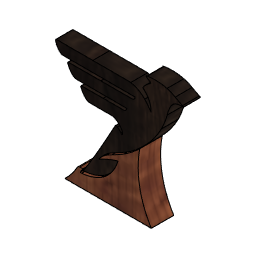
BlackSwiftDeskLogo v10 (Autodesk Fusion 360 design; units mm, degrees)
Autodesk Fusion 360 part; units mm, degrees
sketch "Sketch1" plane through (0, 0, 0) normal (0, 1, 0) x (1, 0, 0)
  spline S0 degree 3 poles (28.812599, -0.914385) (28.812599, -1.007661) (29.30972, -1.834065) (29.917311, -2.750838) knots 0 0 0 0 1 1 1 1
  spline S1 degree 3 poles (29.917311, -2.750838) (36.944588, -13.354057) (46.936102, -30.456433) (58.618766, -51.878822) knots 0 0 0 0 1 1 1 1
  spline S2 degree 3 poles (58.618766, -51.878822) (60.219164, -54.813461) (61.65408, -57.379058) (61.807463, -57.580155) knots 0 0 0 0 1 1 1 1
  spline S3 degree 3 poles (61.807463, -57.580155) (62.243331, -58.151604) (62.6887, -58.094845) (63.845395, -57.320437) knots 0 0 0 0 1 1 1 1
  spline S4 degree 3 poles (63.845395, -57.320437) (64.951702, -56.579755) (66.160509, -55.405523) (67.347976, -53.918028) knots 0 0 0 0 1 1 1 1
  spline S5 degree 3 poles (67.347976, -53.918028) (68.302152, -52.722769) (68.569408, -52.552013) (68.881908, -52.937928) knots 0 0 0 0 1 1 1 1
  spline S6 degree 3 poles (68.881908, -52.937928) (69.341546, -53.505563) (69.008645, -55.565192) (68.194272, -57.192261) knots 0 0 0 0 1 1 1 1
  spline S7 degree 3 poles (68.194272, -57.192261) (67.571278, -58.436976) (66.865745, -59.388616) (65.693126, -60.565893) knots 0 0 0 0 1 1 1 1
  spline S8 degree 3 poles (65.693126, -60.565893) (63.643539, -62.623611) (61.536026, -63.942213) (59.43194, -64.483299) knots 0 0 0 0 1 1 1 1
  spline S9 degree 3 poles (59.43194, -64.483299) (58.739509, -64.661363) (57.820927, -64.673156) (47.446235, -64.637132) knots 0 0 0 0 1 1 1 1
  spline S10 degree 3 poles (47.446235, -64.637132) (36.109744, -64.597772) (34.64539, -64.636087) (33.594249, -64.998073) knots 0 0 0 0 1 1 1 1
  spline S11 degree 3 poles (33.594249, -64.998073) (32.71821, -65.299894) (31.855594, -65.916002) (30.696252, -67.067923) knots 0 0 0 0 1 1 1 1
  spline S12 degree 3 poles (30.696252, -67.067923) (29.044949, -68.708652) (27.40767, -71.223347) (26.483234, -73.538694) knots 0 0 0 0 1 1 1 1
  spline S13 degree 3 poles (26.483234, -73.538694) (26.080684, -74.546929) (26.054861, -74.963611) (26.376872, -75.25504) knots 0 0 0 0 1 1 1 1
  spline S14 degree 3 poles (26.376872, -75.25504) (26.605076, -75.461575) (27.181933, -75.468375) (49.063672, -75.522586) knots 0 0 0 0 1 1 1 1
  line L0 (49.063672, -75.522586) -> (71.516311, -75.57821)
  line L1 (71.516311, -75.57821) -> (71.87243, -75.911946)
  spline S15 degree 3 poles (71.87243, -75.911946) (72.373465, -76.381488) (73.310826, -77.836591) (73.310826, -78.144823) knots 0 0 0 0 1 1 1 1
  spline S16 degree 3 poles (73.310826, -78.144823) (73.310826, -78.286466) (73.199567, -78.480283) (73.063583, -78.57553) knots 0 0 0 0 1 1 1 1
  spline S17 degree 3 poles (73.063583, -78.57553) (72.841591, -78.731021) (70.208488, -78.749104) (47.282424, -78.752587) knots 0 0 0 0 1 1 1 1
  spline S18 degree 3 poles (47.282424, -78.752587) (25.94621, -78.755716) (21.60542, -78.781964) (20.878127, -78.911613) knots 0 0 0 0 1 1 1 1
  spline S19 degree 3 poles (20.878127, -78.911613) (18.537316, -79.328857) (16.127566, -81.699245) (14.031978, -85.645935) knots 0 0 0 0 1 1 1 1
  spline S20 degree 3 poles (14.031978, -85.645935) (12.729457, -88.099011) (12.388433, -89.429148) (12.986959, -89.721938) knots 0 0 0 0 1 1 1 1
  spline S21 degree 3 poles (12.986959, -89.721938) (13.094562, -89.774576) (28.25081, -89.842673) (46.667514, -89.873265) knots 0 0 0 0 1 1 1 1
  spline S22 degree 3 poles (46.667514, -89.873265) (73.988945, -89.918649) (80.199445, -89.955709) (80.407863, -90.074607) knots 0 0 0 0 1 1 1 1
  spline S23 degree 3 poles (80.407863, -90.074607) (80.695616, -90.238763) (81.565868, -91.378616) (81.893942, -92.021069) knots 0 0 0 0 1 1 1 1
  spline S24 degree 3 poles (81.893942, -92.021069) (82.160264, -92.542607) (82.084297, -92.821555) (81.633093, -92.978844) knots 0 0 0 0 1 1 1 1
  spline S25 degree 3 poles (81.633093, -92.978844) (81.387485, -93.064463) (70.631073, -93.099389) (44.504993, -93.099389) knots 0 0 0 0 1 1 1 1
  spline S26 degree 3 poles (44.504993, -93.099389) (3.876362, -93.099389) (7.079301, -93.041478) (5.789219, -93.799384) knots 0 0 0 0 1 1 1 1
  spline S27 degree 3 poles (5.789219, -93.799384) (4.940553, -94.297963) (3.299284, -95.96935) (2.48931, -97.15985) knots 0 0 0 0 1 1 1 1
  spline S28 degree 3 poles (2.48931, -97.15985) (1.193036, -99.065112) (0.103075, -101.631647) (0.094025, -102.800034) knots 0 0 0 0 1 1 1 1
  spline S29 degree 3 poles (0.094025, -102.800034) (0.090443, -103.262371) (0.141743, -103.415042) (0.381101, -103.654396) knots 0 0 0 0 1 1 1 1
  line L2 (0.381101, -103.654396) -> (0.672538, -103.94583)
  line L3 (0.672538, -103.94583) -> (38.465688, -103.94583)
  spline S30 degree 3 poles (38.465688, -103.94583) (74.521314, -103.94583) (76.315092, -103.936495) (77.482534, -103.742926) knots 0 0 0 0 1 1 1 1
  spline S31 degree 3 poles (77.482534, -103.742926) (83.17461, -102.799111) (87.481522, -100.516999) (91.89345, -96.106981) knots 0 0 0 0 1 1 1 1
  spline S32 degree 3 poles (91.89345, -96.106981) (94.083858, -93.917523) (95.823661, -91.737445) (97.489688, -89.094547) knots 0 0 0 0 1 1 1 1
  line L4 (97.489688, -89.094547) -> (98.366273, -87.703977)
  line L5 (98.366273, -87.703977) -> (98.305674, -89.650774)
  spline S33 degree 3 poles (98.305674, -89.650774) (98.239918, -91.763348) (98.039913, -92.960782) (97.43434, -94.867524) knots 0 0 0 0 1 1 1 1
  spline S34 degree 3 poles (97.43434, -94.867524) (97.05087, -96.074941) (96.056162, -98.221095) (95.340677, -99.384761) knots 0 0 0 0 1 1 1 1
  spline S35 degree 3 poles (95.340677, -99.384761) (94.230244, -101.190765) (92.524316, -103.150251) (90.91543, -104.467741) knots 0 0 0 0 1 1 1 1
  spline S36 degree 3 poles (90.91543, -104.467741) (90.275302, -104.991935) (90.108897, -105.190363) (90.108897, -105.429509) knots 0 0 0 0 1 1 1 1
  spline S37 degree 3 poles (90.108897, -105.429509) (90.108897, -106.16981) (91.997399, -108.567541) (93.735112, -110.033524) knots 0 0 0 0 1 1 1 1
  spline S38 degree 3 poles (93.735112, -110.033524) (94.222711, -110.444874) (95.270794, -111.221163) (96.064182, -111.758612) knots 0 0 0 0 1 1 1 1
  spline S39 degree 3 poles (96.064182, -111.758612) (97.206454, -112.532395) (97.551062, -112.826473) (97.71977, -113.171449) knots 0 0 0 0 1 1 1 1
  spline S40 degree 3 poles (97.71977, -113.171449) (97.929662, -113.600668) (97.929662, -113.612985) (97.71977, -114.005009) knots 0 0 0 0 1 1 1 1
  spline S41 degree 3 poles (97.71977, -114.005009) (97.54598, -114.329584) (97.285577, -114.515665) (96.306698, -115.014762) knots 0 0 0 0 1 1 1 1
  spline S42 degree 3 poles (96.306698, -115.014762) (95.039089, -115.661068) (94.193281, -116.31074) (93.658715, -117.048689) knots 0 0 0 0 1 1 1 1
  spline S43 degree 3 poles (93.658715, -117.048689) (93.117943, -117.795204) (93.162979, -117.844139) (94.586522, -118.05692) knots 0 0 0 0 1 1 1 1
  spline S44 degree 3 poles (94.586522, -118.05692) (101.519329, -119.09318) (108.735231, -118.782906) (114.86716, -117.184877) knots 0 0 0 0 1 1 1 1
  spline S45 degree 3 poles (114.86716, -117.184877) (117.554906, -116.484431) (119.695907, -115.590846) (123.298495, -113.665903) knots 0 0 0 0 1 1 1 1
  spline S46 degree 3 poles (123.298495, -113.665903) (127.961824, -111.174193) (129.500391, -110.372518) (130.744363, -109.78622) knots 0 0 0 0 1 1 1 1
  spline S47 degree 3 poles (130.744363, -109.78622) (131.458373, -109.449702) (132.043895, -109.144521) (132.045518, -109.10804) knots 0 0 0 0 1 1 1 1
  spline S48 degree 3 poles (132.045518, -109.10804) (132.047258, -109.071559) (131.287841, -109.007388) (130.358188, -108.965437) knots 0 0 0 0 1 1 1 1
  spline S49 degree 3 poles (130.358188, -108.965437) (124.388559, -108.696058) (121.480194, -107.39743) (119.240974, -104.001451) knots 0 0 0 0 1 1 1 1
  spline S50 degree 3 poles (119.240974, -104.001451) (117.657667, -101.600224) (116.596502, -98.956061) (115.040811, -93.535774) knots 0 0 0 0 1 1 1 1
  spline S51 degree 3 poles (115.040811, -93.535774) (113.32995, -87.574855) (111.543148, -83.000167) (109.026252, -78.136858) knots 0 0 0 0 1 1 1 1
  spline S52 degree 3 poles (109.026252, -78.136858) (104.535546, -69.459641) (98.796243, -61.728751) (91.22576, -54.159483) knots 0 0 0 0 1 1 1 1
  spline S53 degree 3 poles (91.22576, -54.159483) (85.617623, -48.552238) (79.732979, -43.799887) (73.340409, -39.715556) knots 0 0 0 0 1 1 1 1
  spline S54 degree 3 poles (73.340409, -39.715556) (70.30336, -37.775133) (67.906625, -36.437854) (60.851314, -32.747182) knots 0 0 0 0 1 1 1 1
  spline S55 degree 3 poles (60.851314, -32.747182) (57.635155, -31.064785) (56.324494, -30.311792) (54.677187, -29.200059) knots 0 0 0 0 1 1 1 1
  spline S56 degree 3 poles (54.677187, -29.200059) (51.971909, -27.37431) (49.870008, -25.48514) (48.476813, -23.627214) knots 0 0 0 0 1 1 1 1
  spline S57 degree 3 poles (48.476813, -23.627214) (47.732466, -22.634575) (47.07678, -21.511506) (47.180841, -21.40744) knots 0 0 0 0 1 1 1 1
  spline S58 degree 3 poles (47.180841, -21.40744) (47.215665, -21.37261) (47.690109, -21.60197) (48.235162, -21.917117) knots 0 0 0 0 1 1 1 1
  spline S59 degree 3 poles (48.235162, -21.917117) (52.504268, -24.385507) (58.551397, -27.044152) (64.046471, -28.868649) knots 0 0 0 0 1 1 1 1
  spline S60 degree 3 poles (64.046471, -28.868649) (66.31813, -29.622889) (66.858579, -29.77155) (66.858579, -29.642166) knots 0 0 0 0 1 1 1 1
  spline S61 degree 3 poles (66.858579, -29.642166) (66.858579, -29.459655) (65.725346, -26.393405) (65.272588, -25.350849) knots 0 0 0 0 1 1 1 1
  spline S62 degree 3 poles (65.272588, -25.350849) (63.047403, -20.227007) (60.46569, -16.387494) (56.741138, -12.662942) knots 0 0 0 0 1 1 1 1
  spline S63 degree 3 poles (56.741138, -12.662942) (54.272096, -10.193894) (52.293622, -8.639115) (49.369116, -6.869617) knots 0 0 0 0 1 1 1 1
  spline S64 degree 3 poles (49.369116, -6.869617) (43.741178, -3.464391) (36.717991, -1.281855) (29.897239, -0.818488) knots 0 0 0 0 1 1 1 1
  spline S65 degree 3 poles (29.897239, -0.818488) (28.967337, -0.75531) (28.812594, -0.768996) (28.812599, -0.914385) knots 0 0 0 0 1 1 1 1
extrude "Extrude1" add sketch "Sketch1" along normal blind 17.31645 makes body 1
sketch "Sketch2" plane through (0, 17.31645, 0) normal (0, 1, 0) x (-1, 0, 0)
  spline S0 degree 3 poles (-29.897239, 0.818488) (-28.967337, 0.75531) (-28.812594, 0.768996) (-28.812599, 0.914385) knots 0 0 0 0 1 1 1 1
  spline S1 degree 3 poles (-28.812599, 0.914385) (-28.812599, 1.007661) (-29.30972, 1.834065) (-29.917311, 2.750838) knots 0 0 0 0 1 1 1 1
  spline S2 degree 3 poles (-29.917311, 2.750838) (-36.944588, 13.354057) (-46.936102, 30.456433) (-58.618766, 51.878822) knots 0 0 0 0 1 1 1 1
  spline S3 degree 3 poles (-58.618766, 51.878822) (-60.219164, 54.813461) (-61.65408, 57.379058) (-61.807463, 57.580155) knots 0 0 0 0 1 1 1 1
  spline S4 degree 3 poles (-61.807463, 57.580155) (-62.243331, 58.151604) (-62.6887, 58.094845) (-63.845395, 57.320437) knots 0 0 0 0 1 1 1 1
  spline S5 degree 3 poles (-63.845395, 57.320437) (-64.951702, 56.579755) (-66.160509, 55.405523) (-67.347976, 53.918028) knots 0 0 0 0 1 1 1 1
  spline S6 degree 3 poles (-67.347976, 53.918028) (-68.302152, 52.722769) (-68.569408, 52.552013) (-68.881908, 52.937928) knots 0 0 0 0 1 1 1 1
  spline S7 degree 3 poles (-68.881908, 52.937928) (-69.341546, 53.505563) (-69.008645, 55.565192) (-68.194272, 57.192261) knots 0 0 0 0 1 1 1 1
  spline S8 degree 3 poles (-68.194272, 57.192261) (-67.571278, 58.436976) (-66.865745, 59.388616) (-65.693126, 60.565893) knots 0 0 0 0 1 1 1 1
  spline S9 degree 3 poles (-65.693126, 60.565893) (-63.643539, 62.623611) (-61.536026, 63.942213) (-59.43194, 64.483299) knots 0 0 0 0 1 1 1 1
  spline S10 degree 3 poles (-59.43194, 64.483299) (-58.739509, 64.661363) (-57.820927, 64.673156) (-47.446235, 64.637132) knots 0 0 0 0 1 1 1 1
  spline S11 degree 3 poles (-47.446235, 64.637132) (-36.109744, 64.597772) (-34.64539, 64.636087) (-33.594249, 64.998073) knots 0 0 0 0 1 1 1 1
  spline S12 degree 3 poles (-33.594249, 64.998073) (-32.71821, 65.299894) (-31.855594, 65.916002) (-30.696252, 67.067923) knots 0 0 0 0 1 1 1 1
  spline S13 degree 3 poles (-30.696252, 67.067923) (-29.044949, 68.708652) (-27.40767, 71.223347) (-26.483234, 73.538694) knots 0 0 0 0 1 1 1 1
  spline S14 degree 3 poles (-26.483234, 73.538694) (-26.080684, 74.546929) (-26.054861, 74.963611) (-26.376872, 75.25504) knots 0 0 0 0 1 1 1 1
  spline S15 degree 3 poles (-26.376872, 75.25504) (-26.605076, 75.461575) (-27.181933, 75.468375) (-49.063672, 75.522586) knots 0 0 0 0 1 1 1 1
  line L0 (-49.063672, 75.522586) -> (-71.516311, 75.57821)
  line L1 (-71.516311, 75.57821) -> (-71.87243, 75.911946)
  spline S16 degree 3 poles (-71.87243, 75.911946) (-72.373465, 76.381488) (-73.310826, 77.836591) (-73.310826, 78.144823) knots 0 0 0 0 1 1 1 1
  spline S17 degree 3 poles (-73.310826, 78.144823) (-73.310826, 78.286466) (-73.199567, 78.480283) (-73.063583, 78.57553) knots 0 0 0 0 1 1 1 1
  spline S18 degree 3 poles (-73.063583, 78.57553) (-72.841591, 78.731021) (-70.208488, 78.749104) (-47.282424, 78.752587) knots 0 0 0 0 1 1 1 1
  spline S19 degree 3 poles (-47.282424, 78.752587) (-25.94621, 78.755716) (-21.60542, 78.781964) (-20.878127, 78.911613) knots 0 0 0 0 1 1 1 1
  spline S20 degree 3 poles (-20.878127, 78.911613) (-18.537316, 79.328857) (-16.127566, 81.699245) (-14.031978, 85.645935) knots 0 0 0 0 1 1 1 1
  spline S21 degree 3 poles (-14.031978, 85.645935) (-12.729457, 88.099011) (-12.388433, 89.429148) (-12.986959, 89.721938) knots 0 0 0 0 1 1 1 1
  spline S22 degree 3 poles (-12.986959, 89.721938) (-13.094562, 89.774576) (-28.25081, 89.842673) (-46.667514, 89.873265) knots 0 0 0 0 1 1 1 1
  spline S23 degree 3 poles (-46.667514, 89.873265) (-73.988945, 89.918649) (-80.199445, 89.955709) (-80.407863, 90.074607) knots 0 0 0 0 1 1 1 1
  spline S24 degree 3 poles (-80.407863, 90.074607) (-80.695616, 90.238763) (-81.565868, 91.378616) (-81.893942, 92.021069) knots 0 0 0 0 1 1 1 1
  spline S25 degree 3 poles (-81.893942, 92.021069) (-82.160264, 92.542607) (-82.084297, 92.821555) (-81.633093, 92.978844) knots 0 0 0 0 1 1 1 1
  spline S26 degree 3 poles (-81.633093, 92.978844) (-81.387485, 93.064463) (-70.631073, 93.099389) (-44.504993, 93.099389) knots 0 0 0 0 1 1 1 1
  spline S27 degree 3 poles (-44.504993, 93.099389) (-3.876362, 93.099389) (-7.079301, 93.041478) (-5.789219, 93.799384) knots 0 0 0 0 1 1 1 1
  spline S28 degree 3 poles (-5.789219, 93.799384) (-4.940553, 94.297963) (-3.299284, 95.96935) (-2.48931, 97.15985) knots 0 0 0 0 1 1 1 1
  spline S29 degree 3 poles (-2.48931, 97.15985) (-1.193036, 99.065112) (-0.103075, 101.631647) (-0.094025, 102.800034) knots 0 0 0 0 1 1 1 1
  spline S30 degree 3 poles (-0.094025, 102.800034) (-0.090443, 103.262371) (-0.141743, 103.415042) (-0.381101, 103.654396) knots 0 0 0 0 1 1 1 1
  line L2 (-0.381101, 103.654396) -> (-0.672538, 103.94583)
  line L3 (-0.672538, 103.94583) -> (-38.465688, 103.94583)
  spline S31 degree 3 poles (-38.465688, 103.94583) (-74.521314, 103.94583) (-76.315092, 103.936495) (-77.482534, 103.742926) knots 0 0 0 0 1 1 1 1
  spline S32 degree 3 poles (-77.482534, 103.742926) (-83.17461, 102.799111) (-87.481522, 100.516999) (-91.89345, 96.106981) knots 0 0 0 0 1 1 1 1
  spline S33 degree 3 poles (-91.89345, 96.106981) (-94.083858, 93.917523) (-95.823661, 91.737445) (-97.489688, 89.094547) knots 0 0 0 0 1 1 1 1
  line L4 (-97.489688, 89.094547) -> (-98.366273, 87.703977)
  line L5 (-98.366273, 87.703977) -> (-98.305674, 89.650774)
  spline S34 degree 3 poles (-98.305674, 89.650774) (-98.239918, 91.763348) (-98.039913, 92.960782) (-97.43434, 94.867524) knots 0 0 0 0 1 1 1 1
  spline S35 degree 3 poles (-97.43434, 94.867524) (-97.05087, 96.074941) (-96.056162, 98.221095) (-95.340677, 99.384761) knots 0 0 0 0 1 1 1 1
  spline S36 degree 3 poles (-95.340677, 99.384761) (-94.230244, 101.190765) (-92.524316, 103.150251) (-90.91543, 104.467741) knots 0 0 0 0 1 1 1 1
  spline S37 degree 3 poles (-90.91543, 104.467741) (-90.275302, 104.991935) (-90.108897, 105.190363) (-90.108897, 105.429509) knots 0 0 0 0 1 1 1 1
  spline S38 degree 3 poles (-90.108897, 105.429509) (-90.108897, 106.16981) (-91.997399, 108.567541) (-93.735112, 110.033524) knots 0 0 0 0 1 1 1 1
  spline S39 degree 3 poles (-93.735112, 110.033524) (-94.222711, 110.444874) (-95.270794, 111.221163) (-96.064182, 111.758612) knots 0 0 0 0 1 1 1 1
  spline S40 degree 3 poles (-96.064182, 111.758612) (-97.206454, 112.532395) (-97.551062, 112.826473) (-97.71977, 113.171449) knots 0 0 0 0 1 1 1 1
  spline S41 degree 3 poles (-97.71977, 113.171449) (-97.929662, 113.600668) (-97.929662, 113.612985) (-97.71977, 114.005009) knots 0 0 0 0 1 1 1 1
  spline S42 degree 3 poles (-97.71977, 114.005009) (-97.54598, 114.329584) (-97.285577, 114.515665) (-96.306698, 115.014762) knots 0 0 0 0 1 1 1 1
  spline S43 degree 3 poles (-96.306698, 115.014762) (-95.039089, 115.661068) (-94.193281, 116.31074) (-93.658715, 117.048689) knots 0 0 0 0 1 1 1 1
  spline S44 degree 3 poles (-93.658715, 117.048689) (-93.117943, 117.795204) (-93.162979, 117.844139) (-94.586522, 118.05692) knots 0 0 0 0 1 1 1 1
  spline S45 degree 3 poles (-94.586522, 118.05692) (-101.519329, 119.09318) (-108.735231, 118.782906) (-114.86716, 117.184877) knots 0 0 0 0 1 1 1 1
  spline S46 degree 3 poles (-114.86716, 117.184877) (-117.554906, 116.484431) (-119.695907, 115.590846) (-123.298495, 113.665903) knots 0 0 0 0 1 1 1 1
  spline S47 degree 3 poles (-123.298495, 113.665903) (-127.961824, 111.174193) (-129.500391, 110.372518) (-130.744363, 109.78622) knots 0 0 0 0 1 1 1 1
  spline S48 degree 3 poles (-130.744363, 109.78622) (-131.458373, 109.449702) (-132.043895, 109.144521) (-132.045518, 109.10804) knots 0 0 0 0 1 1 1 1
  spline S49 degree 3 poles (-132.045518, 109.10804) (-132.047258, 109.071559) (-131.287841, 109.007388) (-130.358188, 108.965437) knots 0 0 0 0 1 1 1 1
  spline S50 degree 3 poles (-130.358188, 108.965437) (-124.388559, 108.696058) (-121.480194, 107.39743) (-119.240974, 104.001451) knots 0 0 0 0 1 1 1 1
  spline S51 degree 3 poles (-119.240974, 104.001451) (-117.657667, 101.600224) (-116.596502, 98.956061) (-115.040811, 93.535774) knots 0 0 0 0 1 1 1 1
  spline S52 degree 3 poles (-115.040811, 93.535774) (-113.32995, 87.574855) (-111.543148, 83.000167) (-109.026252, 78.136858) knots 0 0 0 0 1 1 1 1
  spline S53 degree 3 poles (-109.026252, 78.136858) (-104.535546, 69.459641) (-98.796243, 61.728751) (-91.22576, 54.159483) knots 0 0 0 0 1 1 1 1
  spline S54 degree 3 poles (-91.22576, 54.159483) (-85.617623, 48.552238) (-79.732979, 43.799887) (-73.340409, 39.715556) knots 0 0 0 0 1 1 1 1
  spline S55 degree 3 poles (-73.340409, 39.715556) (-70.30336, 37.775133) (-67.906625, 36.437854) (-60.851314, 32.747182) knots 0 0 0 0 1 1 1 1
  spline S56 degree 3 poles (-60.851314, 32.747182) (-57.635155, 31.064785) (-56.324494, 30.311792) (-54.677187, 29.200059) knots 0 0 0 0 1 1 1 1
  spline S57 degree 3 poles (-54.677187, 29.200059) (-51.971909, 27.37431) (-49.870008, 25.48514) (-48.476813, 23.627214) knots 0 0 0 0 1 1 1 1
  spline S58 degree 3 poles (-48.476813, 23.627214) (-47.732466, 22.634575) (-47.07678, 21.511506) (-47.180841, 21.40744) knots 0 0 0 0 1 1 1 1
  spline S59 degree 3 poles (-47.180841, 21.40744) (-47.215665, 21.37261) (-47.690109, 21.60197) (-48.235162, 21.917117) knots 0 0 0 0 1 1 1 1
  spline S60 degree 3 poles (-48.235162, 21.917117) (-52.504268, 24.385507) (-58.551397, 27.044152) (-64.046471, 28.868649) knots 0 0 0 0 1 1 1 1
  spline S61 degree 3 poles (-64.046471, 28.868649) (-66.31813, 29.622889) (-66.858579, 29.77155) (-66.858579, 29.642166) knots 0 0 0 0 1 1 1 1
  spline S62 degree 3 poles (-66.858579, 29.642166) (-66.858579, 29.459655) (-65.725346, 26.393405) (-65.272588, 25.350849) knots 0 0 0 0 1 1 1 1
  spline S63 degree 3 poles (-65.272588, 25.350849) (-63.047403, 20.227007) (-60.46569, 16.387494) (-56.741138, 12.662942) knots 0 0 0 0 1 1 1 1
  spline S64 degree 3 poles (-56.741138, 12.662942) (-54.272096, 10.193894) (-52.293622, 8.639115) (-49.369116, 6.869617) knots 0 0 0 0 1 1 1 1
  spline S65 degree 3 poles (-49.369116, 6.869617) (-43.741178, 3.464391) (-36.717991, 1.281855) (-29.897239, 0.818488) knots 0 0 0 0 1 1 1 1
  spline S66 degree 3 poles (-54.819275, 28.98952) (-52.130775, 27.175094) (-50.049238, 25.300774) (-48.680026, 23.474832) knots 0 0 0 0 1 1 1 1
  spline S67 degree 3 poles (-48.680026, 23.474831) (-48.351639, 23.036904) (-48.039267, 22.570778) (-47.806786, 22.185331) (-47.738553, 22.072203) (-47.677357, 21.966324) (-47.6245, 21.87003) knots 0 0 0 0 0.44853488 0.44853488 0.44853488 0.58017901 0.58017901 0.58017901 0.58017901
  spline S68 degree 3 poles (-47.6245, 21.87003) (-47.769513, 21.9459) (-47.935172, 22.037066) (-48.108023, 22.137007) knots 0.67751209 0.67751209 0.67751209 0.67751209 1 1 1 1
  spline S69 degree 3 poles (-48.108023, 22.137007) (-52.398689, 24.617863) (-58.454215, 27.27952) (-63.966434, 29.109709) knots 0 0 0 0 1 1 1 1
  spline S70 degree 3 poles (-63.966434, 29.109709) (-65.103244, 29.487154) (-65.806247, 29.713175) (-66.237032, 29.83167) (-66.452424, 29.890918) (-66.595554, 29.92442) (-66.716533, 29.934989) (-66.797589, 29.94207) (-66.882928, 29.969194) (-67.009734, 29.863245) (-67.07219, 29.811061) (-67.112579, 29.711193) (-67.112579, 29.642166) knots 0 0 0 0 0.5 0.5 0.5 0.75 0.75 0.75 0.91750073 0.91750073 0.91750073 1 1 1 1
  spline S71 degree 3 poles (-67.112579, 29.642166) (-67.112579, 29.559951) (-67.100915, 29.546999) (-67.089711, 29.504284) (-67.031152, 29.281042) (-66.861209, 28.794546) (-66.641738, 28.18985) (-66.272943, 27.173729) (-65.776816, 25.874271) (-65.505566, 25.249672) knots 0 0 0 0 0.06662832 0.06662832 0.06662832 0.41485124 0.41485124 0.41485124 1 1 1 1
  spline S72 degree 3 poles (-65.505566, 25.249671) (-63.270255, 20.102512) (-60.665513, 16.228107) (-56.920744, 12.483337) knots 0 0 0 0 1 1 1 1
  spline S73 degree 3 poles (-56.920744, 12.483337) (-54.441427, 10.004015) (-52.438083, 8.429647) (-49.500605, 6.6523) knots 0 0 0 0 1 1 1 1
  spline S74 degree 3 poles (-49.500605, 6.6523) (-43.833718, 3.223509) (-36.777255, 1.031296) (-29.914455, 0.565072) knots 0 0 0 0 1 1 1 1
  spline S75 degree 3 poles (-29.914455, 0.565072) (-29.392306, 0.529597) (-29.122791, 0.511306) (-28.917281, 0.543155) (-28.812124, 0.559452) (-28.681794, 0.601726) (-28.607774, 0.726193) (-28.567619, 0.793717) (-28.558597, 0.863877) (-28.558599, 0.914394) knots 0 0 0 0 0.55888101 0.55888101 0.55888101 0.84485718 0.84485718 0.84485718 1 1 1 1
  spline S76 degree 3 poles (-28.558599, 0.914394) (-28.558599, 1.020176) (-28.579584, 1.030229) (-28.594686, 1.066288) (-28.659473, 1.220985) (-28.797153, 1.455661) (-28.998333, 1.784767) (-29.191645, 2.101002) (-29.437914, 2.487272) (-29.705589, 2.891157) knots 0 0 0 0 0.10624268 0.10624268 0.10624268 0.5620338 0.5620338 0.5620338 1 1 1 1
  spline S77 degree 3 poles (-29.705589, 2.891157) (-36.724632, 13.481954) (-46.715046, 30.581598) (-58.39577, 52.000433) knots 0 0 0 0 1 1 1 1
  spline S78 degree 3 poles (-58.39577, 52.000433) (-59.19635, 53.46845) (-59.955487, 54.844071) (-60.534062, 55.878552) (-60.824862, 56.398498) (-61.069988, 56.832164) (-61.252285, 57.148821) (-61.384112, 57.377811) (-61.482054, 57.544113) (-61.544737, 57.643779) (-61.567833, 57.680502) (-61.583949, 57.705937) (-61.605503, 57.734195) knots 0 0 0 0 0.5 0.5 0.5 0.75130759 0.75130759 0.75130759 0.93303985 0.93303985 0.93303985 1 1 1 1
  spline S79 degree 3 poles (-61.605505, 57.734197) (-61.832511, 58.031816) (-62.138438, 58.231837) (-62.498796, 58.214821) (-62.918483, 58.195005) (-63.353457, 57.955459) (-63.986703, 57.531501) knots 0 0 0 0 0.46197121 0.46197121 0.46197121 1 1 1 1
  spline S80 degree 3 poles (-63.986704, 57.5315) (-65.125059, 56.769362) (-66.347241, 55.578738) (-67.546481, 54.076495) knots 0 0 0 0 1 1 1 1
  spline S81 degree 3 poles (-67.546481, 54.076495) (-68.032619, 53.467528) (-68.351423, 53.133926) (-68.504629, 53.041432) (-68.594494, 52.987177) (-68.573766, 53.000318) (-68.592782, 53.009983) (-68.604506, 53.015943) (-68.639054, 53.041638) (-68.68451, 53.097773) knots 0 0 0 0 0.51328728 0.51328728 0.51328728 0.81436357 0.81436357 0.81436357 1 1 1 1
  spline S82 degree 3 poles (-68.68451, 53.097773) (-68.777399, 53.212487) (-68.867071, 53.634932) (-68.820237, 54.186331) (-68.749699, 55.016798) (-68.440927, 56.131965) (-67.967134, 57.078576) knots 0 0 0 0 0.39902517 0.39902517 0.39902517 1 1 1 1
  spline S83 degree 3 poles (-67.967134, 57.078576) (-67.355302, 58.30099) (-66.673436, 59.221764) (-65.513165, 60.386644) knots 0 0 0 0 1 1 1 1
  spline S84 degree 3 poles (-65.513165, 60.386644) (-63.486729, 62.42112) (-61.415988, 63.710818) (-59.36868, 64.237302) knots 0 0 0 0 1 1 1 1
  spline S85 degree 3 poles (-59.36868, 64.237302) (-58.992486, 64.334044) (-58.539064, 64.380827) (-56.129668, 64.394846) (-54.423593, 64.404773) (-51.747859, 64.398067) (-47.447117, 64.383133) knots 0 0 0 0 0.58544856 0.58544856 0.58544856 1 1 1 1
  spline S86 degree 3 poles (-47.447117, 64.383133) (-38.728574, 64.352863) (-35.859798, 64.364965) (-34.472767, 64.544108) (-34.056175, 64.597913) (-33.768988, 64.669258) (-33.511545, 64.757915) (-33.511524, 64.757922) (-33.511503, 64.757929) (-33.511482, 64.757936) knots 0 0 0 0 0.76902493 0.76902493 0.76902493 1 1 1 1.00001992 1.00001992 1.00001992 1.00001992
  spline S87 degree 3 poles (-33.511482, 64.757936) (-32.583356, 65.07771) (-31.689119, 65.72335) (-30.517225, 66.887742) knots 0.0000106 0.0000106 0.0000106 0.0000106 1 1 1 1
  spline S88 degree 3 poles (-30.517225, 66.887742) (-28.83342, 68.560765) (-27.186589, 71.092065) (-26.247342, 73.44451) knots 0 0 0 0 1 1 1 1
  spline S89 degree 3 poles (-26.247341, 73.444511) (-25.941948, 74.209405) (-25.809946, 74.680108) (-25.960467, 75.087579) (-26.012074, 75.227282) (-26.100136, 75.347163) (-26.206432, 75.443365) knots 0 0 0 0 0.74468206 0.74468206 0.74468206 1 1 1 1
  spline S90 degree 3 poles (-26.206432, 75.443365) (-26.264241, 75.495685) (-26.38192, 75.557689) (-26.528155, 75.585197) (-26.910418, 75.657106) (-27.749461, 75.684008) (-30.430858, 75.708562) (-33.53795, 75.737013) (-39.085614, 75.751867) (-49.063042, 75.776585) knots 0 0 0 0 0.15053202 0.15053202 0.15053202 0.54403033 0.54403033 0.54403033 1 1 1 1
  line L6 (-49.063042, 75.776585) -> (-71.415629, 75.831961)
  line L7 (-71.415629, 75.831961) -> (-71.69874, 76.097278)
  spline S91 degree 3 poles (-71.698744, 76.097282) (-71.906569, 76.292044) (-72.259998, 76.754895) (-72.546106, 77.195686) (-72.730328, 77.479506) (-72.891871, 77.75951) (-72.982229, 77.953289) (-73.027418, 78.050198) (-73.053809, 78.133008) (-73.056625, 78.148528) knots 0 0 0 0 0.48862959 0.48862959 0.48862959 0.80325171 0.80325171 0.80325171 0.96059418 0.96059418 0.96059418 0.96059418
  spline S92 degree 3 poles (-73.056625, 78.148528) (-73.054448, 78.17286) (-72.996418, 78.298925) (-72.940033, 78.349684) (-72.937865, 78.351635) (-72.935729, 78.353499) (-72.933633, 78.35527) knots 0.06071009 0.06071009 0.06071009 0.06071009 0.88348328 0.88348328 0.88348328 0.91510906 0.91510906 0.91510906 0.91510906
  spline S93 degree 3 poles (-72.933633, 78.35527) (-72.887945, 78.366289) (-72.68876, 78.391361) (-72.323594, 78.407671) (-70.621999, 78.48367) (-65.019229, 78.495893) (-47.282385, 78.498587) knots 0.06031267 0.06031267 0.06031267 0.06031267 0.22634149 0.22634149 0.22634149 1 1 1 1
  spline S94 degree 3 poles (-47.282385, 78.498587) (-36.228979, 78.500208) (-29.736933, 78.508029) (-25.943945, 78.533232) (-23.210779, 78.551392) (-21.88336, 78.578051) (-21.243891, 78.619445) (-21.05778, 78.631492) (-20.930611, 78.644253) (-20.833551, 78.661556) knots 0 0 0 0 0.51805358 0.51805358 0.51805358 0.8913547 0.8913547 0.8913547 1 1 1 1
  spline S95 degree 3 poles (-20.833551, 78.661556) (-18.358778, 79.102678) (-15.921297, 81.5461) (-13.807641, 85.526818) knots 0 0 0 0 1 1 1 1
  spline S96 degree 3 poles (-13.807641, 85.526818) (-13.094885, 86.869171) (-12.662201, 87.878428) (-12.508277, 88.611595) (-12.406104, 89.09826) (-12.410905, 89.495045) (-12.646952, 89.773249) (-12.709753, 89.847266) (-12.788454, 89.907595) (-12.875345, 89.950101) knots 0 0 0 0 0.54336463 0.54336463 0.54336463 0.90404107 0.90404107 0.90404107 1 1 1 1
  spline S97 degree 3 poles (-12.875345, 89.950101) (-12.948043, 89.985664) (-12.945124, 89.973003) (-12.956554, 89.974661) (-13.010765, 89.982528) (-13.036381, 89.98139) (-13.101898, 89.98366) (-13.64543, 90.002489) (-15.803957, 90.021689) (-19.166036, 90.040794) (-25.288244, 90.075585) (-35.3635, 90.108489) (-46.667092, 90.127265) knots 0 0 0 0 0.00856581 0.00856581 0.00856581 0.04919415 0.04919415 0.04919415 0.3862447 0.3862447 0.3862447 1 1 1 1
  spline S98 degree 3 poles (-46.667092, 90.127265) (-60.011902, 90.149432) (-68.320243, 90.169615) (-73.351801, 90.198312) (-75.86758, 90.21266) (-77.564346, 90.229146) (-78.660506, 90.249031) (-79.338772, 90.261335) (-79.788009, 90.27505) (-80.054059, 90.289929) (-80.177213, 90.296816) (-80.26581, 90.304864) (-80.303647, 90.310163) knots 0 0 0 0 0.48844043 0.48844043 0.48844043 0.73266064 0.73266064 0.73266064 0.88377548 0.88377548 0.88377548 0.95372631 0.95372631 0.95372631 0.95372631
  spline S99 degree 3 poles (-80.303647, 90.310163) (-80.350066, 90.345281) (-80.461573, 90.452769) (-80.579543, 90.586897) (-80.940308, 90.997076) (-81.452837, 91.71577) (-81.66773, 92.136586) knots 0.05159173 0.05159173 0.05159173 0.05159173 0.28529727 0.28529727 0.28529727 1 1 1 1
  spline S100 degree 3 poles (-81.66773, 92.136586) (-81.802094, 92.39971) (-81.803685, 92.536199) (-81.781512, 92.586943) (-81.7646, 92.625648) (-81.717244, 92.677557) (-81.567112, 92.732693) knots 0 0 0 0 0.55812729 0.55812729 0.55812729 0.98383913 0.98383913 0.98383913 0.98383913
  spline S101 degree 3 poles (-81.567112, 92.732693) (-81.537123, 92.735873) (-81.427198, 92.742571) (-81.275878, 92.747692) (-79.843086, 92.79618) (-73.820015, 92.825441) (-61.949912, 92.837926) (-57.130128, 92.842995) (-51.344199, 92.845389) (-44.504993, 92.845389) knots 0.02542544 0.02542544 0.02542544 0.02542544 0.0935141 0.0935141 0.0935141 0.73822076 0.73822076 0.73822076 1 1 1 1
  spline S102 degree 3 poles (-44.504993, 92.845389) (-23.022913, 92.845389) (-13.798261, 92.829043) (-9.671166, 92.926045) (-7.331043, 92.981046) (-6.62767, 93.059466) (-6.199625, 93.243812) (-5.954842, 93.349233) (-5.855433, 93.465895) (-5.660558, 93.580381) knots 0 0 0 0 0.52874552 0.52874552 0.52874552 0.82855193 0.82855193 0.82855193 1 1 1 1
  spline S103 degree 3 poles (-5.660558, 93.580381) (-4.993796, 93.972094) (-4.004952, 94.918029) (-3.172378, 95.876531) (-2.832303, 96.268042) (-2.522199, 96.659967) (-2.279306, 97.016971) knots 0 0 0 0 0.70999431 0.70999431 0.70999431 1 1 1 1
  spline S104 degree 3 poles (-2.279306, 97.016971) (-1.333721, 98.406791) (-0.504136, 100.123239) (-0.098671, 101.444625) (0.06132, 101.966026) (0.157067, 102.423605) (0.159968, 102.798067) knots 0 0 0 0 0.71705824 0.71705824 0.71705824 1 1 1 1
  spline S105 degree 3 poles (0.159968, 102.798067) (0.162788, 103.162082) (0.123973, 103.416839) (-0.029877, 103.635166) (-0.079555, 103.705665) (-0.136885, 103.769391) (-0.201498, 103.834003) knots 0 0 0 0 0.75591329 0.75591329 0.75591329 1 1 1 1
  line L8 (-0.201501, 103.834006) -> (-0.567329, 104.19983)
  line L9 (-0.567329, 104.19983) -> (-38.465695, 104.19983)
  spline S106 degree 3 poles (-38.465688, 104.19983) (-63.347649, 104.19983) (-71.909342, 104.195505) (-75.220722, 104.128961) (-76.707759, 104.099078) (-77.149856, 104.055554) (-77.524082, 103.993505) knots 0 0 0 0 0.69009843 0.69009843 0.69009843 1 1 1 1
  spline S107 degree 3 poles (-77.524083, 103.993505) (-83.260945, 103.042264) (-87.63362, 100.724099) (-92.073016, 96.286625) knots 0 0 0 0 1 1 1 1
  spline S108 degree 3 poles (-92.073016, 96.286625) (-94.275486, 94.08511) (-96.029594, 91.887073) (-97.704558, 89.229997) knots 0 0 0 0 1 1 1 1
  line L10 (-97.704555, 89.230002) -> (-98.083353, 88.629096)
  line L11 (-98.083353, 88.629096) -> (-98.051797, 89.642872)
  spline S109 degree 3 poles (-98.051797, 89.642872) (-97.986446, 91.742421) (-97.793426, 92.897759) (-97.192256, 94.790639) knots 0 0 0 0 1 1 1 1
  spline S110 degree 3 poles (-97.192256, 94.790639) (-96.82086, 95.96004) (-95.821822, 98.117281) (-95.124305, 99.251723) knots 0 0 0 0 1 1 1 1
  spline S111 degree 3 poles (-95.124305, 99.251723) (-94.03173, 101.028682) (-92.335971, 102.976187) (-90.754505, 104.271224) knots 0 0 0 0 1 1 1 1
  spline S112 degree 3 poles (-90.754504, 104.271224) (-90.258899, 104.677071) (-90.014904, 104.890038) (-89.904257, 105.169485) (-89.870291, 105.255267) (-89.854897, 105.345666) (-89.854897, 105.429509) knots 0 0 0 0 0.76512711 0.76512711 0.76512711 1 1 1 1
  spline S113 degree 3 poles (-89.854897, 105.429509) (-89.854897, 105.74494) (-90.018847, 106.063656) (-90.261679, 106.467545) (-90.921309, 107.564675) (-92.275606, 109.134558) (-93.571329, 110.227665) knots 0 0 0 0 0.26907672 0.26907672 0.26907672 1 1 1 1
  spline S114 degree 3 poles (-93.571329, 110.227666) (-94.07566, 110.653131) (-95.120309, 111.426015) (-95.921728, 111.968904) knots 0 0 0 0 1 1 1 1
  spline S115 degree 3 poles (-95.921729, 111.968905) (-96.96114, 112.673009) (-97.307964, 112.969641) (-97.454009, 113.213697) (-97.467745, 113.236651) (-97.480094, 113.259522) (-97.491594, 113.283036) knots 0 0 0 0 0.91403319 0.91403319 0.91403319 1 1 1 1
  spline S116 degree 3 poles (-97.491594, 113.283036) (-97.598274, 113.501191) (-97.623624, 113.58167) (-97.623175, 113.60351) (-97.622745, 113.624467) (-97.598113, 113.694108) (-97.495845, 113.885118) knots 0 0 0 0 0.51032178 0.51032178 0.51032178 1 1 1 1
  spline S117 degree 3 poles (-97.495845, 113.885118) (-97.389425, 114.083872) (-97.27338, 114.198606) (-96.80271, 114.464371) (-96.640855, 114.555763) (-96.440137, 114.661616) (-96.191323, 114.788478) knots 0 0 0 0 0.7441137 0.7441137 0.7441137 1 1 1 1
  spline S118 degree 3 poles (-96.191323, 114.788478) (-94.903084, 115.445302) (-94.020705, 116.116005) (-93.453015, 116.899681) knots 0 0 0 0 1 1 1 1
  spline S119 degree 3 poles (-93.453015, 116.899681) (-93.277529, 117.141933) (-93.145295, 117.303916) (-93.097185, 117.525875) (-93.066271, 117.668501) (-93.124606, 117.866403) (-93.242664, 117.966738) (-93.446949, 118.140355) (-93.694739, 118.170103) (-94.098185, 118.237748) (-94.231389, 118.260082) (-94.380987, 118.28302) (-94.548973, 118.308129) knots 0 0 0 0 0.32034979 0.32034979 0.32034979 0.5261993 0.5261993 0.5261993 0.88239596 0.88239596 0.88239596 1 1 1 1
  spline S120 degree 3 poles (-94.548973, 118.308129) (-101.514596, 119.349295) (-108.759994, 119.038936) (-114.931215, 117.430668) knots 0 0 0 0 1 1 1 1
  spline S121 degree 3 poles (-114.931215, 117.430668) (-117.638121, 116.725228) (-119.807533, 115.819186) (-123.418197, 113.889929) knots 0 0 0 0 1 1 1 1
  spline S122 degree 3 poles (-123.418197, 113.889929) (-128.081017, 111.39849) (-129.616391, 110.598643) (-130.852651, 110.01598) knots 0 0 0 0 1 1 1 1
  spline S123 degree 3 poles (-130.852651, 110.01598) (-131.21222, 109.846512) (-131.539189, 109.685102) (-131.779484, 109.559857) (-131.899632, 109.497235) (-131.997599, 109.44403) (-132.070749, 109.400987) (-132.107323, 109.379466) (-132.137038, 109.361191) (-132.165675, 109.340817) (-132.182481, 109.328861) (-132.19766, 109.319191) (-132.224381, 109.2912) (-132.243155, 109.271534) (-132.292906, 109.257959) (-132.29923, 109.120141) knots 0 0 0 0 0.5 0.5 0.5 0.75 0.75 0.75 0.875 0.875 0.875 0.94835905 0.94835905 0.94835905 0.99989924 0.99989924 0.99989924 0.99989924
  spline S124 degree 3 poles (-132.29923, 109.120141) (-132.305107, 108.996921) (-132.230512, 108.927771) (-132.197171, 108.902305) (-132.113654, 108.838514) (-132.100255, 108.85332) (-132.073855, 108.84688) (-131.960881, 108.819324) (-131.815338, 108.806446) (-131.58763, 108.786977) (-131.275453, 108.760286) (-130.844803, 108.733137) (-130.369638, 108.711695) knots 0 0 0 0 0.03457717 0.03457717 0.03457717 0.12119151 0.12119151 0.12119151 0.49184746 0.49184746 0.49184746 1 1 1 1
  spline S125 degree 3 poles (-130.369638, 108.711695) (-125.245609, 108.480474) (-122.4738, 107.507553) (-120.396013, 105.114284) (-120.066511, 104.73475) (-119.75415, 104.318312) (-119.453025, 103.86163) knots 0 0 0 0 0.86312292 0.86312292 0.86312292 1 1 1 1
  spline S126 degree 3 poles (-119.453025, 103.86163) (-117.88818, 101.4884) (-116.838239, 98.877604) (-115.284954, 93.465702) knots 0 0 0 0 1 1 1 1
  spline S127 degree 3 poles (-115.284954, 93.465702) (-113.570662, 87.492831) (-111.776059, 82.897587) (-109.251833, 78.020113) knots 0 0 0 0 1 1 1 1
  spline S128 degree 3 poles (-109.251833, 78.020113) (-104.748829, 69.319133) (-98.991595, 61.56489) (-91.40535, 53.979863) knots 0 0 0 0 1 1 1 1
  spline S129 degree 3 poles (-91.40535, 53.979863) (-85.785134, 48.36054) (-79.885468, 43.595898) (-73.477165, 39.501514) knots 0 0 0 0 1 1 1 1
  spline S130 degree 3 poles (-73.477165, 39.501514) (-70.433642, 37.556955) (-68.025753, 36.213517) (-60.969047, 32.522116) knots 0 0 0 0 1 1 1 1
  spline S131 degree 3 poles (-60.969047, 32.522116) (-57.755357, 30.84101) (-56.458882, 30.096055) (-54.819275, 28.98952) knots 0 0 0 0 1 1 1 1
  line L12 (-12.7, -12.7) -> (-101.6, -12.7)
  arc A0 (-101.6, -12.7) -> (-89.733, 52.340958) centre (-178.929861, 35.012234) ccw
  arc A1 (-25.556843, 3.790757) -> (-12.7, -12.7) centre (36.431581, 38.862145) ccw
  line L13 (-27.767546, 5.08) -> (-31.138635, 5.08)
  arc A2 (-25.556843, 3.790757) -> (-27.767546, 5.08) centre (-27.767546, 2.54) ccw
  dimension "d3" = 0.254
  dimension "d5" = 88.9
  dimension "d9" = 2.54
  constraint horizontal L12
  constraint horizontal L13
  constraint tangent A1 A2
  constraint tangent L13 A2
  measures "d5" distance of L12.start L12.end
  measures "d9" radius of A2
extrude "Extrude2" add sketch "Sketch2" against normal blind 20.202525 separate body contours S66 S67 S68 S69 S70 S71 S72 S73 S74 S75 S76 S77 S129 S130 S131 L12 A0 A1 L13 A2 picked at (-50.813815, -7.826102) makes body 2
move_face "OffsetFaces1" offset 2.886075 1 faces at (50.813815, 17.31645, -7.826102) on bodies 2
scale "Scale1" factor 1.1 about (91.22576, 0, 54.159483) bodies 2 1
